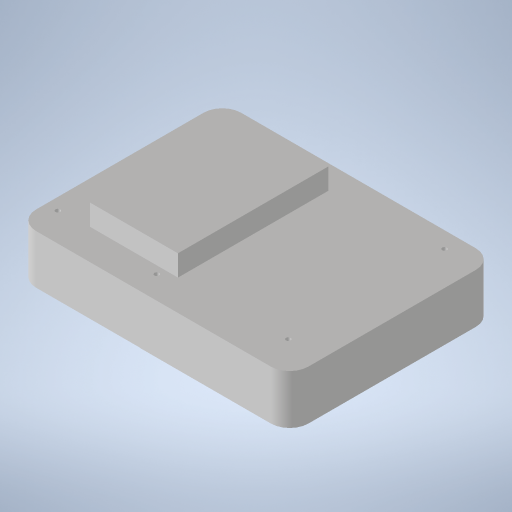
# Autodesk Inventor part: Isdt
Saved by Autodesk Inventor 2023.1 (Build 271208000, 208)
## iProperties
Created: 2022-09-09
Part Number: Isdt
Material: Generisch
Document SubType Name: Modeling
Designer: Rama
Density: 1 g/cm^3
Appearance: Vorgabe
Author: Rama
Autodesk Inventor part; units mm, degrees
ref_plane "YZ Plane" through (0, 0, 0) normal (1, 0, 0) x (0, 1, 0)
ref_plane "XZ Plane" through (0, 0, 0) normal (0, 1, 0) x (-1, 0, 0)
ref_plane "XY Plane" through (0, 0, 0) normal (0, 0, 1) x (1, 0, 0)
sketch "Skizze1" plane through (0, 0, 0) normal (0, 1, 0) x (-1, 0, 0)
  line L0 (50.25, 43.85) -> (-50.25, 43.85)
  line L1 (-58.25, 35.85) -> (-58.25, -35.85)
  line L2 (-50.25, -43.85) -> (50.25, -43.85)
  line L3 (58.25, -35.85) -> (58.25, 35.85)
  line L4 (58.25, 43.85) -> (-58.25, -43.85) construction
  line L5 (-58.25, 43.85) -> (58.25, -43.85) construction
  arc A0 (58.25, 35.85) -> (50.25, 43.85) centre (50.25, 35.85) ccw
  arc A1 (50.25, -43.85) -> (58.25, -35.85) centre (50.25, -35.85) ccw
  arc A2 (-58.25, -35.85) -> (-50.25, -43.85) centre (-50.25, -35.85) ccw
  arc A3 (-50.25, 43.85) -> (-58.25, 35.85) centre (-50.25, 35.85) ccw
  point P0 (0, 0)
  dimension "d0" = 116.5
  dimension "d1" = 87.7
  dimension "d2" = 8
  constraints: 12 end point, 8 point on circle, 8 point on line, 8 tangent, 4 centre point, 3 equal radius, 2 midpoint, 2 parallel, 1 horizontal, 1 perpendicular
  measures "d0" distance of L5.end L4.end
  measures "d1" distance of L4.end L5.start
  measures "d2" radius of A0
extrude "Extrusion1" add sketch "Skizze1" along normal blind 21
sketch "Skizze2" plane through (0, 0, 0) normal (0, -1, 0) x (1, 0, 0)
  arc A0 (58.25, 35.85) -> (50.25, 43.85) centre (50.25, 35.85) ccw projected
  line L0 (-50.25, 43.85) -> (50.25, 43.85) projected
  arc A1 (-50.25, 43.85) -> (-58.25, 35.85) centre (-50.25, 35.85) ccw projected
  line L1 (-58.25, -35.85) -> (-58.25, 35.85) projected
  arc A2 (-58.25, -35.85) -> (-50.25, -43.85) centre (-50.25, -35.85) ccw projected
  line L2 (50.25, -43.85) -> (-50.25, -43.85) projected
  arc A3 (50.25, -43.85) -> (58.25, -35.85) centre (50.25, -35.85) ccw projected
  line L3 (58.25, 35.85) -> (58.25, -35.85) projected
  line L4 (50.25, -43.85) -> (-50.25, -43.85) projected
  line L5 (-5.75, -43.85) -> (-5.75, 43.85)
  point P0 (0, 0)
  dimension "d5" = 64
  constraints: 2 end point, 2 point on line, 1 perpendicular
  measures "d5" distance between parallel lines of L5 L3
extrude "Extrusion2" add sketch "Skizze2" along normal blind 0.1 contours L3 A3 L2 L5 L0 A0
sketch "Skizze3" plane through (0, 21, 0) normal (0, 1, 0) x (1, 0, 0)
  line L0 (-40.25, -30.75) -> (-2.65, -30.75)
  line L1 (-2.65, -30.75) -> (-2.65, 33.55)
  line L2 (-2.65, 33.55) -> (-40.25, 33.55)
  line L3 (-40.25, 33.55) -> (-40.25, -30.75)
  line L4 (-40.25, -30.75) -> (-2.65, 33.55) construction
  line L5 (-2.65, -30.75) -> (-40.25, 33.55) construction
  line L6 (-50.25, -43.85) -> (50.25, -43.85) projected
  line L7 (50.25, 43.85) -> (-50.25, 43.85) projected
  line L8 (-58.25, 35.85) -> (-58.25, -35.85) projected
  point P0 (0, 0)
  point P1 (-21.45, 1.4)
  dimension "d8" = 37.6
  dimension "d9" = 64.3
  dimension "d10" = 13.1
  dimension "d11" = 10.3
  dimension "d12" = 18
  constraints: 12 end point, 2 midpoint, 2 parallel, 1 horizontal, 1 perpendicular
  measures "d8" distance of L2.end L1.end
  measures "d9" distance of L1.end L0.end
  measures "d10" distance between parallel lines of L0 L6
  measures "d11" distance between parallel lines of L7 L2
  measures "d12" distance between parallel lines of L3 L8
extrude "Extrusion3" add sketch "Skizze3" along normal blind 9
sketch "Skizze4" plane through (0, -0.1, 0) normal (0, -1, 0) x (1, 0, 0)
  line L0 (50.25, 43.85) -> (-5.75, 43.85) projected
  line L1 (-5.75, 43.85) -> (-5.75, -43.85) projected
  line L2 (-5.75, -43.85) -> (50.25, -43.85) projected
  arc A0 (50.25, -43.85) -> (58.25, -35.85) centre (50.25, -35.85) ccw projected
  line L3 (58.25, -35.85) -> (58.25, 35.85) projected
  arc A1 (58.25, 35.85) -> (50.25, 43.85) centre (50.25, 35.85) ccw projected
  line L4 (-5.75, -43.85) -> (-5.75, 43.85) projected
  line L5 (-50.25, 43.85) -> (-5.75, 43.85) projected
  arc A2 (-50.25, 43.85) -> (-58.25, 35.85) centre (-50.25, 35.85) ccw projected
  line L6 (-58.25, -35.85) -> (-58.25, 35.85) projected
  arc A3 (-58.25, -35.85) -> (-50.25, -43.85) centre (-50.25, -35.85) ccw projected
  line L7 (-5.75, -43.85) -> (-50.25, -43.85) projected
  circle A4 centre (43.75, -36.9) radius 1.1
  circle A5 centre (43.75, 29.95) radius 1.1
  circle A6 centre (-11.95, -35.9681) radius 1.1
  circle A7 centre (-8.45, 34.0319) radius 1.1
  circle A8 centre (-47.95, -34.8429) radius 1.1
  circle A9 centre (-53.15, 31.6571) radius 1.1
  point P0 (0, 0)
  dimension "d15" = 2.2
  dimension "d16" = 2.2
  dimension "d17" = 2.2
  dimension "d18" = 2.2
  dimension "d19" = 2.2
  dimension "d20" = 2.2
  dimension "d21" = 0
  dimension "d22" = 66.85
  dimension "d23" = 70
  dimension "d24" = 66.5
  dimension "d25" = 52.2
  dimension "d26" = 44.7
  dimension "d27" = 36
  dimension "d28" = 55.7
  dimension "d29" = 118.7
  dimension "d30" = 112.2809
  dimension "d31" = 86.3
  dimension "d32" = 88.0691
  dimension "d33" = 79.3976
  dimension "d34" = 13.9
  dimension "d35" = 6.95
  dimension "d36" = 14.5
  dimension "d37" = 9.8181
  dimension "d38" = 7.8819
  dimension "d39" = 9.0071
  dimension "d40" = 12.1929
  dimension "d41" = 5.1
  constraints: 6 centre point
  measures "d15" diameter of A4
  measures "d16" diameter of A5
  measures "d17" diameter of A6
  measures "d18" diameter of A7
  measures "d19" diameter of A8
  measures "d20" diameter of A9
  measures "d21" horizontal distance of A5.centre A4.centre
  measures "d22" distance of A5.centre A4.centre
  measures "d23" vertical distance of A7.centre A6.centre
  measures "d24" vertical distance of A9.centre A8.centre
  measures "d25" horizontal distance of A7.centre A5.centre
  measures "d26" horizontal distance of A9.centre A7.centre
  measures "d27" horizontal distance of A8.centre A6.centre
  measures "d28" horizontal distance of A6.centre A4.centre
  measures "d29" distance of A4.centre A9.centre
  measures "d30" distance of A8.centre A5.centre
  measures "d31" distance of A6.centre A5.centre
  measures "d32" distance of A7.centre A4.centre
  measures "d33" distance of A8.centre A7.centre
  measures "d34" distance from line of L0 A5.centre
  measures "d35" distance from line of L2 A4.centre
  measures "d36" distance from line of A4.centre L3
  measures "d37" distance from line of A7.centre L0
  measures "d38" distance from line of L7 A6.centre
  measures "d39" distance from line of L7 A8.centre
  measures "d40" distance from line of A9.centre L5
  measures "d41" distance from line of A9.centre L6
hole "Bohrung1" at (-11.95, -0.1, -35.9681) at (-47.95, -0.1, -34.8429) at (-53.15, -0.1, 31.6571) at (-8.45, -0.1, 34.0319) at (43.75, -0.1, 29.95) at (43.75, -0.1, -36.9) direction (0, 1, 0) diameter 2 end through all
sketch "Skizze5" plane through (-58.25, 0, -35.85) normal (-1, 0, 0) x (0, 0, 1)
  line L0 (0, 0) -> (71.7, 0) projected
  line L1 (71.7, 0) -> (71.7, 21) projected
  line L2 (0, 21) -> (71.7, 21) projected
  line L3 (0, 0) -> (0, 21) projected
  line L4 (14.13, 18.35) -> (7.13, 18.35)
  line L5 (6.13, 17.35) -> (6.13, 16.05)
  line L6 (7.13, 15.05) -> (14.13, 15.05)
  line L7 (15.13, 16.05) -> (15.13, 17.35)
  arc A0 (15.13, 17.35) -> (14.13, 18.35) centre (14.13, 17.35) ccw
  arc A1 (14.13, 15.05) -> (15.13, 16.05) centre (14.13, 16.05) ccw
  arc A2 (6.13, 16.05) -> (7.13, 15.05) centre (7.13, 16.05) ccw
  arc A3 (7.13, 18.35) -> (6.13, 17.35) centre (7.13, 17.35) ccw
  line L8 (-8, 0) -> (0, 0) projected
  line L9 (0, 0) -> (0, 21) projected
  line L10 (-8, 21) -> (0, 21) projected
  line L11 (-8, 0) -> (-8, 21) projected
  point P0 (35.85, 0)
  point P1 (6.13, 15.05)
  point P2 (6.13, 18.35)
  point P3 (15.13, 15.05)
  point P4 (6.13, 16.7)
  dimension "d49" = 9
  dimension "d50" = 3.3
  dimension "d51" = 1
  dimension "d52" = 15.05
  dimension "d53" = 14.13
  constraints: 8 end point, 8 point on circle, 8 tangent, 6 point on line, 4 centre point, 3 equal radius, 2 parallel, 1 horizontal, 1 midpoint, 1 perpendicular
  measures "d49" distance of point (15.13, 15.05) point (6.13, 15.05)
  measures "d50" distance of point (6.13, 15.05) point (6.13, 18.35)
  measures "d51" radius of A0
  measures "d52" distance between parallel lines of L6 L0
  measures "d53" distance from line of L11 point (6.13, 16.7)
extrude "Extrusion4" cut sketch "Skizze5" against normal blind 6 contours A0 L7 A1 L6 A2 L5 A3 L4
equation "\"d16\" = d15"
equation "\"d17\" = d15"
equation "\"d18\" = d15"
equation "\"d19\" = d15"
equation "\"d20\" = d15"
